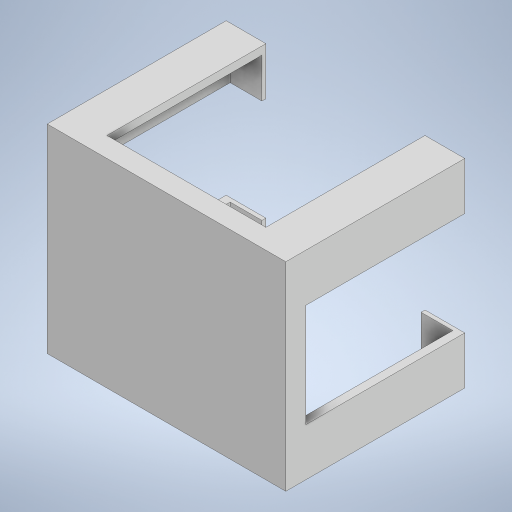
# Autodesk Inventor part: MESA_TALADRADO
Saved by Autodesk Inventor 2024 (Build 280153000, 153)
## iProperties
Created: 2023-05-17
Part Number: MESA_TALADRADO
Material: Genérico
Document SubType Name: Modeling
Designer: sebas
Density: 1 g/cm^3
Appearance: Valor por defecto
Author: sebas
Autodesk Inventor part; units mm, degrees
ref_plane "YZ Plane" through (0, 0, 0) normal (1, 0, 0) x (0, 1, 0)
ref_plane "XZ Plane" through (0, 0, 0) normal (0, 1, 0) x (-1, 0, 0)
ref_plane "XY Plane" through (0, 0, 0) normal (0, 0, 1) x (1, 0, 0)
sketch "Boceto1" plane through (0, 0, 0) normal (0, 0, 1) x (1, 0, 0)
  line L0 (-300, -250) -> (300, -250)
  line L1 (300, -250) -> (300, 250)
  line L2 (300, 250) -> (-300, 250)
  line L3 (-300, 250) -> (-300, -250)
  line L4 (-300, -250) -> (300, 250) construction
  line L5 (300, -250) -> (-300, 250) construction
  line L6 (-300, 250) -> (-200, 250)
  line L7 (-200, 250) -> (-200, 230)
  line L8 (-280, 130) -> (-300, 130)
  line L9 (-300, 130) -> (-300, 250)
  line L10 (-300, 130) -> (-280, 130)
  line L11 (-280, 130) -> (-280, 230)
  line L12 (-280, 230) -> (-200, 230)
  line L13 (0, 0) -> (0, 50)
  line L14 (0, 0) -> (-60, 0)
  line L15 (-300, 250) -> (300, 250)
  line L16 (300, 250) -> (300, -250)
  line L17 (-300, -250) -> (300, 250) construction
  line L18 (300, 250) -> (200, 250)
  line L19 (200, 250) -> (200, 230)
  line L20 (300, 130) -> (300, 250)
  line L21 (280, 130) -> (280, 230)
  line L22 (280, 230) -> (200, 230)
  line L23 (280, 130) -> (300, 130)
  line L24 (300, -250) -> (-300, -250)
  line L25 (-300, -250) -> (-300, 250)
  line L26 (300, 250) -> (-300, -250) construction
  line L27 (-300, -250) -> (-200, -250)
  line L28 (-200, -250) -> (-200, -230)
  line L29 (-280, -130) -> (-300, -130)
  line L30 (-300, -130) -> (-300, -250)
  line L31 (-300, -130) -> (-280, -130)
  line L32 (-280, -130) -> (-280, -230)
  line L33 (-280, -230) -> (-200, -230)
  line L34 (-300, -250) -> (300, -250)
  line L35 (300, -250) -> (200, -250)
  line L36 (200, -250) -> (200, -230)
  line L37 (300, -130) -> (300, -250)
  line L38 (280, -130) -> (280, -230)
  line L39 (280, -230) -> (200, -230)
  line L40 (280, -130) -> (300, -130)
  point P0 (-300, 130)
  point P1 (-300, -130)
  point P2 (-200, -250)
  point P3 (200, -250)
  point P4 (300, -130)
  point P5 (300, 130)
  point P6 (200, 250)
  point P7 (-200, 250)
  dimension "d0" = 600
  dimension "d1" = 500
  dimension "d4" = 20
  dimension "d5" = 100
  dimension "d6" = 60
  dimension "d13" = 20
  constraints: 82 end point, 28 symmetric about line, 4 horizontal, 4 parallel, 4 perpendicular, 2 midpoint, 1 vertical
  measures "d0" distance of L2.end L1.end
  measures "d1" distance of L1.end L0.end
  measures "d4" distance of L8.start L8.end
  measures "d5" distance of L8.start L11.end
  measures "d6" distance of L13.start L14.end
  measures "d13" distance of L6.end L7.end
extrude "Extrusión1" add sketch "Boceto1" along normal blind 50 contours L28 L33 L32 L29 L3 L8 L11 L12 L7 L2 L19 L22 L21 L23 L1 L40 L38 L39 L36 L0
extrude "Extrusión2" add sketch "Boceto1" along normal blind 50 and the other way blind 390 contours L3 L29 L32 L33 L28 L0 | L36 L39 L38 L40 L1 L0 | L3 L2 L7 L12 L11 L8 | L23 L21 L22 L19 L2 L1
sketch "Boceto2" plane through (0, 0, -390) normal (0, 0, -1) x (-1, 0, 0)
  line L0 (280, 230) -> (280, 130) projected
  line L1 (200, 230) -> (280, 230) projected
  line L2 (200, 250) -> (200, 230) projected
  line L3 (-200, 250) -> (200, 250) projected
  line L4 (-200, 230) -> (-200, 250) projected
  line L5 (-280, 230) -> (-200, 230) projected
  line L6 (-280, 130) -> (-280, 230) projected
  line L7 (-300, 130) -> (-280, 130) projected
  line L8 (-300, -130) -> (-300, 130) projected
  line L9 (-280, -130) -> (-300, -130) projected
  line L10 (-280, -230) -> (-280, -130) projected
  line L11 (-200, -230) -> (-280, -230) projected
  line L12 (-200, -250) -> (-200, -230) projected
  line L13 (200, -250) -> (-200, -250) projected
  line L14 (200, -230) -> (200, -250) projected
  line L15 (280, -230) -> (200, -230) projected
  line L16 (280, -130) -> (280, -230) projected
  line L17 (300, -130) -> (280, -130) projected
  line L18 (300, 130) -> (300, -130) projected
  line L19 (280, 130) -> (300, 130) projected
  line L20 (300, 250) -> (300, -250) projected
  line L21 (300, -250) -> (200, -250)
  line L22 (200, -250) -> (200, -130)
  line L23 (200, -130) -> (300, -130)
  line L24 (300, -130) -> (300, -250)
  line L25 (-300, 250) -> (-200, 250)
  line L26 (-200, 250) -> (-200, 130)
  line L27 (-200, 130) -> (-300, 130)
  line L28 (-300, 130) -> (-300, 250)
  line L29 (300, 250) -> (200, 250)
  line L30 (200, 250) -> (200, 130)
  line L31 (200, 130) -> (300, 130)
  line L32 (300, 130) -> (300, 250)
  line L33 (-300, -250) -> (-200, -250)
  line L34 (-200, -250) -> (-200, -130)
  line L35 (-200, -130) -> (-300, -130)
  line L36 (-300, -130) -> (-300, -250)
  point P0 (0, 0)
  constraints: 32 end point, 8 parallel, 6 point on line, 4 horizontal, 4 perpendicular
extrude "Extrusión3" add sketch "Boceto2" along normal blind 10 contours L1 L2 L29 L20 L19 L0 | L0 L31 L30 L1 | L20 L21 L14 L15 L16 L17 | L4 L5 L6 L7 L28 L25 | L16 L15 L22 L23 | L26 L27 L6 L5 | L33 L36 L9 L10 L11 L12 | L11 L10 L35 L34
